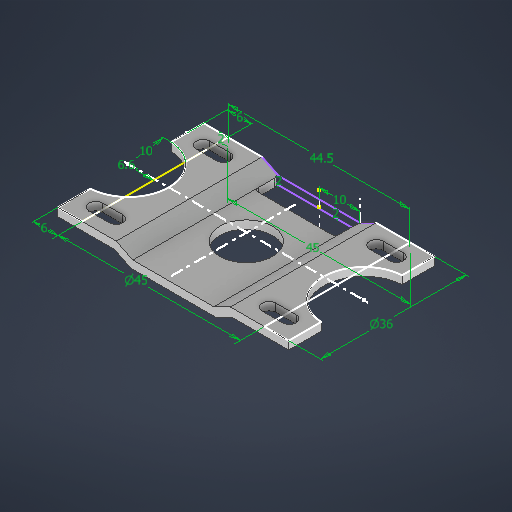
# Autodesk Inventor part: 連接件
Saved by Autodesk Inventor 2025 (Build 290162000, 162)
## iProperties
Created: 2024-01-23
Part Number: 連接件
Material: 一般
Document SubType Name: Modeling
Designer: Justin Tasi
Density: 1 g/cm^3
Appearance: 預設
Author: Justin Tasi
Autodesk Inventor part; units mm, degrees
ref_plane "YZ Plane" through (0, 0, 0) normal (1, 0, 0) x (0, 1, 0)
ref_plane "XZ Plane" through (0, 0, 0) normal (0, 1, 0) x (-1, 0, 0)
ref_plane "XY Plane" through (0, 0, 0) normal (0, 0, 1) x (1, 0, 0)
sketch "草圖1" plane through (0, 0, 0) normal (0, 0, 1) x (1, 0, 0)
  line L0 (-22.5, 3.5874) -> (-14.0953, 3.5874)
  line L1 (-14.0953, 3.5874) -> (-10, 1.5874)
  line L2 (-10, 1.5874) -> (0, 1.5874)
  line L3 (0.691, -0.4126) -> (-10.4623, -0.4126)
  line L4 (-10.4623, -0.4126) -> (-14.5576, 1.5874)
  line L5 (-14.5576, 1.5874) -> (-22.5, 1.5874)
  line L6 (-22.5, 1.5874) -> (-22.5, 3.5874)
  line L7 (0, 2.1547) -> (0, -6.606) construction
  line L8 (22.5, 3.5874) -> (14.0953, 3.5874)
  line L9 (14.0953, 3.5874) -> (10, 1.5874)
  line L10 (10, 1.5874) -> (0, 1.5874)
  line L11 (0.691, -0.4126) -> (10.4623, -0.4126)
  line L12 (10.4623, -0.4126) -> (14.5576, 1.5874)
  line L13 (14.5576, 1.5874) -> (22.5, 1.5874)
  line L14 (22.5, 1.5874) -> (22.5, 3.5874)
  line L15 (-22.25, -3.3995) -> (-22.25, 2.4631)
  line L16 (22.25, -3.2727) -> (22.25, 2.4631)
  line L17 (10, -4.4814) -> (10, 6.978)
  point P0 (0, 0)
  point P1 (-22.25, 1.5321)
  point P2 (22.25, 1.5874)
  point P3 (22.25, 1.5321)
  dimension "d1" = 2
  dimension "d5" = 44.5
  dimension "d9" = 45
  dimension "d32" = 10
  dimension "d36" = 2
  dimension "d46" = 2
  constraints: 36 end point, 6 symmetric about line, 5 vertical, 3 horizontal, 3 parallel, 2 point on line, 1 perpendicular, 1 other
  measures "d1" distance of L5.end L0.start
  measures "d5" distance between parallel lines of L16 L15
  measures "d9" distance between parallel lines of L14 L6
  measures "d32" distance of L9.end L2.end
  measures "d36" distance between parallel lines of L11 L10
  measures "d46" distance between parallel lines of L1 L4
extrude "擠出1" add sketch "草圖1" along normal blind 36
sketch "草圖2" plane through (-22.5, 3.5874, 0) normal (0, 1, 0) x (1, 0, 0)
  point P0 (22.5, 0)
sketch "草圖3" plane through (-22.5, 3.5874, 0) normal (0, 1, 0) x (1, 0, 0)
  line L0 (0, 0) -> (0, -36) projected
  line L1 (0, 0) -> (0, -10.4873)
  line L2 (0, 0) -> (-6, 0)
  line L3 (-6, 0) -> (-6, -8.018)
  line L4 (-6, -36) -> (0, -36)
  line L5 (-6, -27.982) -> (-6, -36)
  line L6 (22.5, -5.8594) -> (22.5, -37.147)
  arc A0 (0, -10.4873) -> (-6, -8.018) centre (-6.6, -18) ccw
  arc A1 (-6, -27.982) -> (0, -10.4873) centre (-6.6, -18) ccw
  line L7 (0, -25.5127) -> (0, -36)
  line L8 (45, 0) -> (45, -36)
  line L9 (45, 0) -> (45, -10.4873)
  line L10 (45, 0) -> (51, 0)
  line L11 (51, 0) -> (51, -8.018)
  line L12 (51, -36) -> (45, -36)
  line L13 (51, -27.982) -> (51, -36)
  arc A2 (51, -8.018) -> (45, -10.4873) centre (51.6, -18) ccw
  arc A3 (45, -10.4873) -> (51, -27.982) centre (51.6, -18) ccw
  line L14 (45, -25.5127) -> (45, -36)
  line L15 (-7.7403, -18) -> (53.0258, -18)
  point P0 (22.5, 0)
  point P1 (45, -25.5127)
  point P2 (-6, -4.009)
  dimension "d13" = 6.6
  dimension "d18" = 45
  dimension "d19" = 6
  dimension "d20" = 6
  dimension "d37" = 10
  dimension "d47" = 36
  constraints: 30 end point, 10 point on circle, 9 symmetric about line, 4 centre point, 4 perpendicular, 2 collinear, 2 horizontal, 1 midpoint, 1 point on line, 1 vertical, 2 other
  measures "d13" distance from line of A0.centre L0
  measures "d18" diameter of L0.end L6
  measures "d19" distance between parallel lines of L5 L0
  measures "d20" distance from line of point (-6, -4.009) L0
  measures "d37" radius of A1
  measures "d47" diameter of L10 L15
extrude "擠出2" add sketch "草圖3" against normal blind 2 contours L8 L10 L11 A2 | A3 L13 L12 L8 | L0 L4 L5 A1 | L0 A0 L3 L2
extrude "擠出3" cut sketch "草圖3" against normal blind 2.5 contours A3 L8 L15 | L15 L8 A3 | A1 L15 L0 | L15 A1 L0
sketch "草圖4" plane through (-14.0953, 3.5874, 36) normal (0, 1, 0) x (1, 0, 0)
  line L0 (-14.4047, 36) -> (-0.4623, 36) projected
  line L1 (-8.1547, 36) -> (-8.1547, -2.5095)
  line L2 (-14.4047, 36) -> (-14.4047, 27.982) projected
  line L3 (28.1906, 0) -> (42.5953, 0) projected
  line L4 (-9.798, 31.25) -> (-4.798, 31.25) construction
  line L5 (-9.798, 29.55) -> (-4.798, 29.55)
  line L6 (-4.798, 32.95) -> (-9.798, 32.95)
  arc A0 (-9.798, 32.95) -> (-9.798, 29.55) centre (-9.798, 31.25) ccw
  arc A1 (-4.798, 29.55) -> (-4.798, 32.95) centre (-4.798, 31.25) ccw
  line L7 (-25.514, 18) -> (67.1526, 18)
  line L8 (14.0953, -5.2274) -> (14.0953, 45.8177)
  circle A2 centre (14.0953, 18) radius 6.5
  line L9 (-9.798, 4.75) -> (-4.798, 4.75) construction
  line L10 (-9.798, 6.45) -> (-4.798, 6.45)
  line L11 (-4.798, 3.05) -> (-9.798, 3.05)
  arc A3 (-9.798, 6.45) -> (-9.798, 3.05) centre (-9.798, 4.75) ccw
  arc A4 (-4.798, 3.05) -> (-4.798, 6.45) centre (-4.798, 4.75) ccw
  line L12 (37.9886, 31.25) -> (32.9886, 31.25) construction
  line L13 (37.9886, 29.55) -> (32.9886, 29.55)
  line L14 (32.9886, 32.95) -> (37.9886, 32.95)
  arc A5 (37.9886, 29.55) -> (37.9886, 32.95) centre (37.9886, 31.25) ccw
  arc A6 (32.9886, 32.95) -> (32.9886, 29.55) centre (32.9886, 31.25) ccw
  arc A7 (32.9886, 6.45) -> (32.9886, 3.05) centre (32.9886, 4.75) ccw
  line L15 (37.9886, 6.45) -> (32.9886, 6.45)
  line L16 (37.9886, 4.75) -> (32.9886, 4.75) construction
  arc A8 (37.9886, 3.05) -> (37.9886, 6.45) centre (37.9886, 4.75) ccw
  line L17 (32.9886, 3.05) -> (37.9886, 3.05)
  point P0 (14.0953, 36)
  point P1 (-7.298, 31.25)
  point P2 (-7.298, 4.75)
  point P3 (35.4886, 31.25)
  point P4 (35.4886, 4.75)
  dimension "d21" = 6.25
  dimension "d33" = 3.4
  dimension "d48" = 36
  dimension "d49" = 13
  dimension "d52" = 26.5
  dimension "d53" = 9.2134
  dimension "d54" = 5
  constraints: 38 end point, 21 symmetric about line, 16 point on circle, 9 centre point, 4 tangent, 3 point on line, 3 vertical, 2 horizontal, 1 midpoint, 1 parallel, 6 other
  measures "d21" distance between parallel lines of L1 L2
  measures "d33" diameter of A1
  measures "d48" diameter of L3 L7
  measures "d49" diameter of A2
  measures "d52" distance between parallel lines of L9 L4
  measures "d53" diameter of L6.end L2
  measures "d54" distance of L6.start L6.end
extrude "擠出4" cut sketch "草圖4" against normal up to surface (4 mm away)
sketch "草圖5" plane through (-10, 1.5874, 0) normal (0, 1, 0) x (1, 0, 0)
  line L0 (-0.4623, 0) -> (20.4623, 0) projected
  line L1 (0, 0) -> (20, 0)
  line L2 (20, 0) -> (20, -6)
  line L3 (20, -6) -> (0, -6)
  line L4 (0, -6) -> (0, 0)
  line L5 (10, -2.0229) -> (10, 3.2313)
  point P0 (10, 0)
  point P1 (20, 0)
  point P2 (20, 0)
  point P3 (10, 0)
  dimension "d38" = 6
  dimension "d42" = 20
  constraints: 10 end point, 2 parallel, 2 point on line, 1 horizontal, 1 midpoint, 1 perpendicular, 1 vertical, 1 other
  measures "d38" distance of L1.end L2.end
  measures "d42" distance of L2.end L3.end
extrude "擠出5" cut sketch "草圖5" against normal up to surface (2 mm away)
fillet "圓角2" radius 1 4 edges at (-10, 0.5874, 0) (10, 0.5874, 0) (-10, 0.5874, 6) (10, 0.5874, 6)
